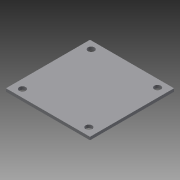
# Autodesk Inventor part: pcb
Saved by Autodesk Inventor 2013 (Build 170138000, 138)
## iProperties
Created: 2014-05-23
Part Number: pcb
Material: Generic
Document SubType Name: Modeling
Designer: balogh
Density: 1 g/cm^3
Author: balogh
Autodesk Inventor part; units mm, degrees
ref_plane "YZ Plane" through (0, 0, 0) normal (1, 0, 0) x (0, 1, 0)
ref_plane "XZ Plane" through (0, 0, 0) normal (0, 1, 0) x (-1, 0, 0)
ref_plane "XY Plane" through (0, 0, 0) normal (0, 0, 1) x (1, 0, 0)
sketch "Sketch1" plane through (0, 0, 0) normal (0, 0, 1) x (1, 0, 0)
  line L0 (-22.5171, -22.5171) -> (22.5171, -22.5171)
  line L1 (22.5171, -22.5171) -> (22.5171, 22.5171)
  line L2 (22.5171, 22.5171) -> (-22.5171, 22.5171)
  line L3 (-22.5171, 22.5171) -> (-22.5171, -22.5171)
  circle A0 centre (18.415, 17.78) radius 1.7526
  circle A1 centre (18.415, -17.78) radius 1.7526
  circle A2 centre (-18.415, -17.78) radius 1.7526
  circle A3 centre (-18.415, 17.78) radius 1.7526
  point P0 (0, 0)
  constraints: 8 end point, 4 centre point, 3 equal radius, 2 perpendicular, 1 parallel
extrude "Extrusion1" add sketch "Sketch1" along normal blind 1.6002
body "Solid1"
